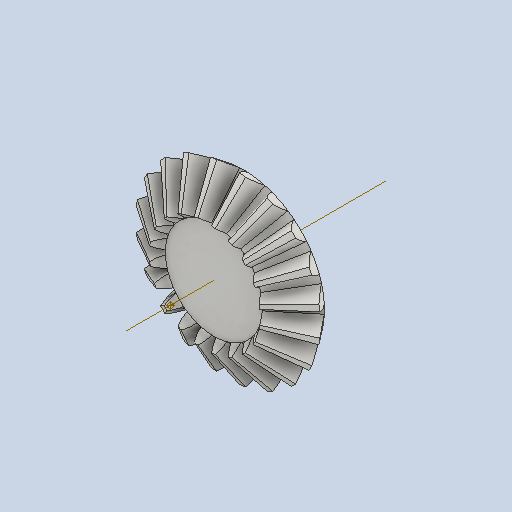
# Autodesk Inventor part: Bevel Gear1
Saved by Autodesk Inventor 2025.2 (Build 292293000, 293)
## iProperties
Created: 2025-01-23
Part Number: Bevel Gear1
Material: Steel, Mild
Document SubType Name: Modeling
Designer: yash3
Categories: <?xml version="1.0" encoding="UTF-16"?> <MemberInstance><Categories><FamilyTemplate><FamilyTemplateParameter ValueType="xs:double" Id="1" ObjectReferenceKey="da_z" ObjectType="kUserParameterObject"/><FamilyTemplateParameter ValueType="xs:double" Id="2" ObjectReferenceKey="da_b" ObjectType="kUserParameterObject"/><FamilyTemplateParameter ValueType="xs:double" Id="3" ObjectReferenceKey="da_beta" ObjectType="kUserParameterObject"/><FamilyTemplateParameter ValueType="xs:double" Id="4" ObjectReferenceKey="da_dae" ObjectType="kUserParameterObject"/><FamilyTemplateParameter ValueType="xs:double" Id="5" ObjectReferenceKey="da_ve" ObjectType="kUserParameterObject"/><FamilyTemplateParameter ValueType="xs:double" Id="6" ObjectReferenceKey="da_omega" ObjectType="kUserParameterObject"/><FamilyTemplateParameter ValueType="xs:string" Id="7" ObjectReferenceKey="EAIAABAAAAAAHwAAAAAAAIAAAAAAAAAA" ObjectType="83914240" SubObjectId="SurfaceGeometry"/></FamilyTemplate><ParamToTemplateMap><ParamToTemplate CategoryParameter="//CategoryParameter[@InternalName='046C89C9-8512-4d59-83FE-43B91F4F132A']" TemplateParameter="1"/><ParamToTemplate CategoryParameter="//CategoryParameter[@InternalName='2552DF32-E462-4b46-AEBF-C6C7768E72AC']" TemplateParameter="2"/><ParamToTemplate CategoryParameter="//CategoryParameter[@InternalName='C9EE641D-15FC-4fae-A226-E94C4372FDD7']" TemplateParameter="3"/><ParamToTemplate><ParamToTemplate CategoryParameter="//CategoryParameter[@InternalName='00B6519A-459B-49c7-AD84-2E56D39A5744']" ConstantValue="0.000000"/></ParamToTemplate><ParamToTemplate><ParamToTemplate CategoryParameter="//CategoryParameter[@InternalName='04B31F0E-C7A6-4894-AA32-9629BEFACF47']" ConstantValue="1.000000"/></ParamToTemplate><ParamToTemplate><ParamToTemplate CategoryParameter="//CategoryParameter[@InternalName='43CBEC2E-7847-49e7-A936-2F7889FCB2D9']" ConstantValue="0.200000"/></ParamToTemplate><ParamToTemplate><ParamToTemplate CategoryParameter="//CategoryParameter[@InternalName='B1EFC894-105D-4ebd-86BF-FA20ED196853']" ConstantValue="0.300000"/></ParamToTemplate><ParamToTemplate><ParamToTemplate CategoryParameter="//CategoryParameter[@InternalName='51175063-3D10-4879-93E8-6246FE8B403D']" ConstantValue="2060000000.000000"/></ParamToTemplate><ParamToTemplate><ParamToTemplate CategoryParameter="//CategoryParameter[@InternalName='A3A52E27-4454-46a9-B0BD-C932399B70AF']" ConstantValue="0.300000"/></ParamToTemplate><ParamToTemplate CategoryParameter="//CategoryParameter[@InternalName='2A200944-5A8C-41ca-B96E-8520D2E510F1']" TemplateParameter="4"/><ParamToTemplate><ParamToTemplate CategoryParameter="//CategoryParameter[@InternalName='1A637F62-92C8-44bc-B81F-10802510B579']" ConstantValue="1.908000"/></ParamToTemplate><ParamToTemplate CategoryParameter="//CategoryParameter[@InternalName='B52DD4BE-6863-48fb-BF58-89EF6F9EC65C']" TemplateParameter="5"/><ParamToTemplate><ParamToTemplate CategoryParameter="//CategoryParameter[@InternalName='3956BFF2-84D2-457d-93C2-9B0613DEBA67']" ConstantValue="0.603000"/></ParamToTemplate><ParamToTemplate CategoryParameter="//CategoryParameter[@InternalName='739CFA02-461B-4bf8-8049-181FCAD8B28F']" TemplateParameter="6"/><ParamToTemplate><ParamToTemplate CategoryParameter="//CategoryParameter[@InternalName='A27E999F-E2CE-4481-8A2A-EBF499C4C3C5']" ConstantValue="0.000000"/></ParamToTemplate><ParamToTemplate><ParamToTemplate CategoryParameter="//CategoryParameter[@InternalName='9E1B4470-B2D3-4ff1-B813-535BB4CDF51A']" ConstantValue="3520000.000000"/></ParamToTemplate><ParamToTemplate><ParamToTemplate CategoryParameter="//CategoryParameter[@InternalName='F8452263-BFF6-458c-9FB1-07C4B99E95CD']" ConstantValue="11400000.000000"/></ParamToTemplate><ParamToTemplate><ParamToTemplate CategoryParameter="//CategoryParameter[@InternalName='3E3BB259-FD49-497f-8171-6EBC954A3479']" ConstantValue="2.000000"/></ParamToTemplate><ParamToTemplate CategoryParameter="//CategoryParameter[@InternalName='27C3BAF2-7550-4e4b-AE2C-0DB134B7D9B7']" TemplateParameter="7"/></ParamToTemplateMap><Category DisplayName="Gear" InternalName="DC85795E-93AB-48d5-8EEE-5A27447B64BD" Mnemonic="Gear"><CategoryParameter DisplayName="z" InternalName="046C89C9-8512-4d59-83FE-43B91F4F132A" Mnemonic="z"/><CategoryParameter DisplayName="b" InternalName="2552DF32-E462-4b46-AEBF-C6C7768E72AC" Mnemonic="b"/><CategoryParameter DisplayName="||b|" InternalName="C9EE641D-15FC-4fae-A226-E94C4372FDD7" Mnemonic="beta"/><CategoryParameter DisplayName="x" InternalName="00B6519A-459B-49c7-AD84-2E56D39A5744" Mnemonic="x"/><CategoryParameter DisplayName="a*" InternalName="04B31F0E-C7A6-4894-AA32-9629BEFACF47" Mnemonic="a"/><CategoryParameter DisplayName="c*" InternalName="43CBEC2E-7847-49e7-A936-2F7889FCB2D9" Mnemonic="c"/><CategoryParameter DisplayName="r|.f|*" InternalName="B1EFC894-105D-4ebd-86BF-FA20ED196853" Mnemonic="rf"/><CategoryParameter DisplayName="E" InternalName="51175063-3D10-4879-93E8-6246FE8B403D" Mnemonic="E"/><CategoryParameter DisplayName="||m|" InternalName="A3A52E27-4454-46a9-B0BD-C932399B70AF" Mnemonic="mi"/><Category DisplayName="BevelGear" InternalName="0C98F69A-0C2B-4791-B2FE-7691BB227E77" Mnemonic="BevelGear"><CategoryParameter DisplayName="d|.ae|" InternalName="2A200944-5A8C-41ca-B96E-8520D2E510F1" Mnemonic="dae"/><CategoryParameter DisplayName="d|.ai|" InternalName="1A637F62-92C8-44bc-B81F-10802510B579" Mnemonic="dai"/><CategoryParameter DisplayName="A|.e|" InternalName="B52DD4BE-6863-48fb-BF58-89EF6F9EC65C" Mnemonic="ve"/><CategoryParameter DisplayName="A|.i|" InternalName="3956BFF2-84D2-457d-93C2-9B0613DEBA67" Mnemonic="vi"/><CategoryParameter DisplayName="||S|" InternalName="739CFA02-461B-4bf8-8049-181FCAD8B28F" Mnemonic="omega"/><CategoryParameter DisplayName="x|.t|" InternalName="A27E999F-E2CE-4481-8A2A-EBF499C4C3C5" Mnemonic="xt"/><CategoryParameter DisplayName="||s||.Flim|" InternalName="9E1B4470-B2D3-4ff1-B813-535BB4CDF51A" Mnemonic="sFlim"/><CategoryParameter DisplayName="||s||.Hlim|" InternalName="F8452263-BFF6-458c-9FB1-07C4B99E95CD" Mnemonic="sHlim"/><CategoryParameter DisplayName="type" InternalName="3E3BB259-FD49-497f-8171-6EBC954A3479" Mnemonic="type"/><CategoryParameter DisplayName="PitchDiameter" InternalName="27C3BAF2-7550-4e4b-AE2C-0DB134B7D9B7" Mnemonic="IDS_PITCHDIAM"/></Category></Category></Categories></MemberInstance>
Mass: 60.9118 g
Surface Area: 34.3074 cm^2
Volume: 7.7496 cm^3
Density: 7.86 g/cm^3
Appearance: Steel
CustomPartVersion: 1
Author: yash3
Autodesk Inventor part; units mm, degrees
ref_plane "Mesh Plane2" through (0, 0, 0) normal (0.9876883, 0.1564345, 0) x (0, 0, 1)
sketch "Teeth Body Sketch" plane through (0, 0, 0) normal (1, 0, 0) x (0, 1, 0)
  line L0 (0, 0) -> (13.92, -12.69) construction
  line L1 (13.92, -12.69) -> (15.9, -10.05)
  line L2 (15.9, -10.05) -> (0, 0) construction
  line L3 (15, -11.25) -> (0, 0) construction
  line L4 (8.352, -7.614) -> (9.54, -6.03)
  line L5 (13.92, -12.69) -> (8.352, -7.614)
  line L6 (15.9, -10.05) -> (9.54, -6.03)
  line L7 (0, -39.386751) -> (0, 6.564458)
  line L8 (0, -11.25) -> (15.9, -11.25) construction
  dimension "d0" = 30
  dimension "d1" = 27.84
  dimension "d2" = 31.8
  dimension "d3" = 7.5
  dimension "d4" = 10.05
  constraints: 16 end point, 4 point on line, 3 perpendicular, 2 collinear, 1 horizontal alignment, 1 vertical alignment
  measures "d0" diameter of L3.start L7
  measures "d1" diameter of L0.end L7
  measures "d2" diameter of L1.end L7
  measures "d3" distance between parallel lines of L1 L4
  measures "d4" vertical distance of L1.end L0.start
revolve "Teeth Body" add sketch "Teeth Body Sketch" angle 360 about axis through (0, 0, 0) along (0, 0, 1)
ref_plane "Tooth Plane" through (0, 15, -11.25) normal (0, -0.8, 0.6) x (1, 0, 0)
sketch "Start Sketch" plane through (0, 15, -11.25) normal (0, -0.8, 0.6) x (1, 0, 0)
  line L0 (0, -23.505131) -> (0, 10.644758)
  arc A0 (-0.581798, -2.196) -> (-2.668261, 2.360199) centre (-9.544236, -3.544417) ccw
  arc A1 (2.668261, 2.360199) -> (0.581798, -2.196) centre (9.544236, -3.544417) ccw
  line L1 (-0.581798, -2.196) -> (0.581798, -2.196)
  arc A2 (2.668261, 2.360199) -> (-2.668261, 2.360199) centre (0, -25) ccw
  dimension "d7" = 9.06331
  dimension "d8" = 9.54424
  dimension "d9" = 21.45558
  dimension "d57" = 27.49
  dimension "d58" = 22.804
  constraints: 6 point on circle, 3 centre point, 3 symmetric about line, 2 end point, 1 coincident, 1 perpendicular, 1 other
  measures "d7" radius of A0
  measures "d8" horizontal distance of point (0, -25) A0.centre
  measures "d9" vertical distance of point (0, -25) A0.centre
  measures "d57" radius of A2
  measures "d58" distance from line of A2.centre L1
sketch "End Sketch" plane through (0, 8.868, -6.651) normal (0, -0.8, 0.6) x (1, 0, 0)
  line L0 (0, -15.35404) -> (0, 6.953444)
  arc A0 (-0.343959, -1.298275) -> (-1.577476, 1.39535) centre (-5.642552, -2.095459) ccw
  arc A1 (1.577476, 1.39535) -> (0.343959, -1.298275) centre (5.642552, -2.095459) ccw
  line L1 (-0.343959, -1.298275) -> (0.343959, -1.298275)
  arc A2 (1.577476, 1.39535) -> (-1.577476, 1.39535) centre (0, -14.78) ccw
  dimension "d12" = 5.35823
  dimension "d15" = 5.64255
  dimension "d16" = 12.68454
  dimension "d59" = 16.25209
  dimension "d60" = 13.48172
  constraints: 6 point on circle, 3 centre point, 3 symmetric about line, 2 end point, 1 coincident, 1 other
  measures "d12" radius of A0
  measures "d15" horizontal distance of A0.centre point (0, -14.78)
  measures "d16" vertical distance of A0.centre point (0, -14.78)
  measures "d59" radius of A2
  measures "d60" distance from line of A2.centre L1
loft "Loft" cut profiles "Start Sketch", "End Sketch"
pattern_circular "Circular Pattern" count 20 over 360 about axis through (0, 0, 0) along (0, 0, 1) of "Loft"
ref_plane "End Plane" through (0, 8.868, -6.651) normal (0, -0.8, 0.6) x (1, 0, 0)
sketch3d "3D Sketch Right"
ref_plane "End Plane Right" through (-2.043164, 8.629421, -6.651) normal (0.1843179, -0.7784773, 0.6) x (0.9730966, 0.2303973, 0)
sketch "End Sketch Right" plane through (-2.043164, 8.629421, -6.651) normal (0.1843179, -0.7784773, 0.6) x (0.9730966, 0.2303973, 0)
  arc A0 (-0.343959, -1.298275) -> (-1.577476, 1.39535) centre (-5.642552, -2.095459) ccw
  line L0 (0, -20.970926) -> (0, 9.95758)
  arc A1 (1.577476, 1.39535) -> (0.343959, -1.298275) centre (5.642552, -2.095459) ccw
  line L1 (-0.343959, -1.298275) -> (0.343959, -1.298275)
  arc A2 (1.577476, 1.39535) -> (-1.577476, 1.39535) centre (0, -14.78) ccw
  dimension "d70" = 5.64255
  dimension "d71" = 12.68454
  dimension "d72" = 5.35823
  dimension "d73" = 13.48172
  dimension "d74" = 16.25209
  constraints: 6 point on circle, 3 centre point, 3 symmetric about line, 2 end point, 1 coincident, 1 perpendicular, 1 other
  measures "d70" horizontal distance of A2.centre A0.centre
  measures "d71" vertical distance of point (0, -14.78) A0.centre
  measures "d72" radius of A0
  measures "d73" distance from line of point (0, -14.78) L1
  measures "d74" radius of A2
feature "Loft Right" [suppressed]
pattern_circular "Circular Pattern Right" [suppressed]
sketch3d "3D Sketch Left"
ref_plane "End Plane Left" through (2.067762, 8.629421, -6.662007) normal (-0.1863493, -0.777694, 0.6003882) x (0.9724716, -0.2330214, 0)
sketch "End Sketch Left" plane through (2.067762, 8.629421, -6.662007) normal (-0.1863493, -0.777694, 0.6003882) x (0.9724716, -0.2330214, 0)
  line L0 (0, -30.712904) -> (0, 13.690181)
  arc A0 (-0.343959, -1.292893) -> (-1.577476, 1.400732) centre (-5.642552, -2.090077) ccw
  arc A1 (1.577476, 1.400732) -> (0.343959, -1.292893) centre (5.642552, -2.090077) ccw
  line L1 (-0.343959, -1.292893) -> (0.343959, -1.292893)
  ellipse E0 centre (0, -4.822243) end of major axis (9.54, -4.822243) minor radius 5.727704
  arc A2 (1.577476, 1.400732) -> (-1.577476, 1.400732) centre (0, -14.774618) ccw
  dimension "d56" = 5.7277
  dimension "d30" = 5.35823
  dimension "d31" = 5.64255
  dimension "d32" = 12.68454
  dimension "d61" = 16.25209
  dimension "d62" = 13.48172
  constraints: 6 point on circle, 3 centre point, 3 symmetric about line, 2 end point, 1 coincident, 2 other
  measures "d30" radius of A0
  measures "d31" horizontal distance of point (0, -14.775) A0.centre
  measures "d32" vertical distance of A0.centre point (0, -14.775)
  measures "d61" radius of A2
  measures "d62" distance from line of point (0, -14.775) L1
feature "Loft Left" [suppressed]
pattern_circular "Circular Pattern Left" [suppressed]
sketch "Body Sketch" plane through (0, 0, 0) normal (1, 0, 0) x (0, 1, 0)
  line L0 (0, -35.037536) -> (0, -19.530831)
  line L1 (13.92, -12.69) -> (8.352, -7.614)
  line L2 (8.352, -7.614) -> (0, -7.614)
  line L3 (13.92, -12.69) -> (0, -12.69)
  constraints: 4 end point, 2 perpendicular, 2 point on line
sketch "Body Sketch outline for Fix Body" plane through (0, 0, 0) normal (1, 0, 0) x (0, 1, 0)
  line L0 (0, -12.69) -> (13.92, -12.69)
  line L1 (0, -7.614) -> (0, -12.69)
  line L2 (8.352, -7.614) -> (0, -7.614)
  line L3 (13.92, -12.69) -> (8.352, -7.614)
revolve "Fix Body" add sketch "Body Sketch outline for Fix Body" angle 360 about axis through (0, 0, 0) along (0, 0, 1)
sketch "Sketch6" plane through (0, 0, 0) normal (1, 0, 0) x (0, 1, 0)
  line L0 (15, -11.25) -> (0, 0)
  line L1 (0, -37.799919) -> (0, 6.299986)
surface revolve "Pitch Diameter" sketch "Sketch6" angle 360 about axis through (0, 0, 0) along (0, 0, 1) shown no curves L0
equation "\"d0\" = da_de"
equation "\"d1\" = da_dfe"
equation "\"d2\" = da_dae"
equation "\"d3\" = da_b"
equation "\"d4\" = da_ve"
equation "\"d7\" = fd_rr"
equation "\"d8\" = fd_x"
equation "\"d9\" = fd_y"
equation "\"d57\" = 0.5 * fd_dva + 0.3 * da_he"
equation "\"d58\" = 0.5 * fd_dva - 1.12 * da_he"
equation "\"da_teethtype\" = 0"
equation "\"da_b\" = 7.5"
equation "\"da_de\" = 30"
equation "\"da_dae\" = 31.8"
equation "\"da_dfe\" = 27.84"
equation "\"da_le\" = 18.75"
equation "\"da_omega\" = 90deg"
equation "\"da_beta\" = 0"
equation "\"da_delta\" = 53.130102deg"
equation "\"da_alpha\" = 20deg"
equation "\"da_he\" = 3.3"
equation "\"da_ve\" = 10.05"
equation "\"da_zv\" = 33.333333"
equation "\"fd_loft\" = da_b + 0.05 * da_he"
equation "\"fd_x\" = fd_x1 + fd_x2"
equation "\"fd_y\" = fd_y1 - fd_y2"
equation "\"fd_dd\" = fd_dva - 0.8 * da_he"
equation "\"d11\" = fd_loft"
equation "\"da_dm\" = 24"
equation "\"da_x\" = 0"
equation "\"da_m\" = 1.5"
equation "\"d50\" = da_omega"
equation "\"fd_rr\" = 9.063306"
equation "\"fd_dva\" = 53"
equation "\"fd_x1\" = 1.190737"
equation "\"fd_x2\" = 8.353499"
equation "\"fd_y1\" = 24.971627"
equation "\"fd_y2\" = 3.516044"
body "Solid1"
body "Srf1"
